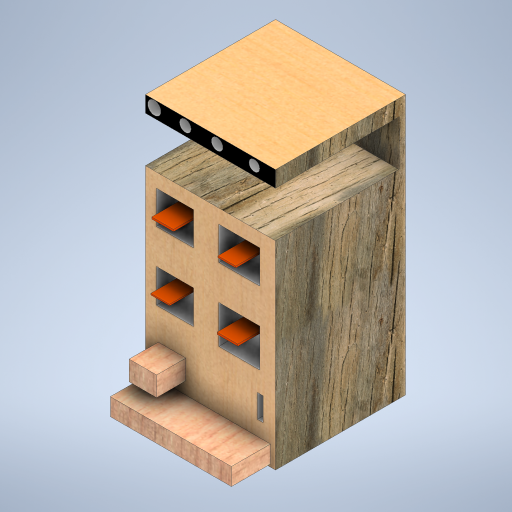
# Autodesk Inventor part: fff
Saved by Autodesk Inventor 2023 (Build 270158000, 158)
## iProperties
Created: 2022-06-05
Part Number: fff
Material: Generic
Document SubType Name: Modeling
Designer: Tushar
Density: 1 g/cm^3
Appearance: Default
Author: Tushar
Autodesk Inventor part; units mm, degrees
ref_plane "YZ Plane" through (0, 0, 0) normal (1, 0, 0) x (0, 1, 0)
ref_plane "XZ Plane" through (0, 0, 0) normal (0, 1, 0) x (-1, 0, 0)
ref_plane "XY Plane" through (0, 0, 0) normal (0, 0, 1) x (1, 0, 0)
sketch "Sketch1" plane through (0, 0, 0) normal (0, 1, 0) x (-1, 0, 0)
  line L0 (17.4506, 75.8516) -> (-84.1494, 75.8516)
  line L1 (-84.1494, 75.8516) -> (-84.1494, -25.7484)
  line L2 (-84.1494, -25.7484) -> (17.4506, -25.7484)
  line L3 (17.4506, -25.7484) -> (17.4506, 75.8516)
  point P0 (0, 0)
  dimension "d0" = 101.6
  dimension "d1" = 101.6
  constraints: 8 end point, 2 parallel, 1 horizontal, 1 perpendicular
  measures "d0" distance of L2.end L0.start
  measures "d1" distance of L1.end L2.end
extrude "Extrusion1" add sketch "Sketch1" along normal blind 203.2
sketch "Sketch2" plane through (-17.4506, 0, 75.8516) normal (0, 0, 1) x (1, 0, 0)
  line L0 (0, 0) -> (0, 203.2) projected
  line L1 (101.6, 0) -> (101.6, 203.2) projected
  line L2 (0, 190.6053) -> (101.6, 190.6053)
  line L3 (101.6, 190.6053) -> (101.6, 155.0988)
  line L4 (101.6, 155.0988) -> (0, 155.0988)
  line L5 (0, 155.0988) -> (0, 190.6053)
  point P0 (17.4506, 0)
  point P1 (0, 155.0988)
  point P2 (101.6, 190.6053)
  constraints: 8 end point, 2 parallel, 2 point on line, 1 horizontal, 1 perpendicular
extrude "Extrusion2" cut sketch "Sketch2" against normal blind 96.52
sketch "Sketch3" plane through (-17.4506, 203.2, 75.8516) normal (0, 0, 1) x (1, 0, 0)
  circle A0 centre (6.9601, -5.4934) radius 5.1747
  circle A1 centre (31.169, -5.4934) radius 4.519
  circle A2 centre (56.0236, -5.4934) radius 4.519
  circle A3 centre (85.0743, -5.4934) radius 4.1962
  point P0 (17.4506, -203.2)
  constraints: 4 centre point
extrude "Extrusion3" cut sketch "Sketch3" against normal blind 8.89
sketch "Sketch4" plane through (-17.4506, 0, 75.8516) normal (0, 0, 1) x (1, 0, 0)
  line L0 (8.574, 144.124) -> (37.6248, 144.124)
  line L1 (37.6248, 144.124) -> (37.6248, 118.3011)
  line L2 (37.6248, 118.3011) -> (8.574, 118.3011)
  line L3 (8.574, 118.3011) -> (8.574, 144.124)
  line L4 (57.3147, 144.124) -> (89.2705, 144.124)
  line L5 (89.2705, 144.124) -> (89.2705, 118.3011)
  line L6 (89.2705, 118.3011) -> (57.3147, 118.3011)
  line L7 (57.3147, 118.3011) -> (57.3147, 144.124)
  line L8 (8.574, 91.1871) -> (37.6248, 91.1871)
  line L9 (37.6248, 91.1871) -> (37.6248, 65.0414)
  line L10 (37.6248, 65.0414) -> (8.574, 65.0414)
  line L11 (8.574, 65.0414) -> (8.574, 91.1871)
  line L12 (57.3147, 91.1871) -> (89.2705, 91.1871)
  line L13 (89.2705, 91.1871) -> (89.2705, 61.4908)
  line L14 (89.2705, 61.4908) -> (57.3147, 61.4908)
  line L15 (57.3147, 61.4908) -> (57.3147, 91.1871)
  point P0 (17.4506, 0)
  constraints: 32 end point, 8 parallel, 7 point on line, 4 horizontal, 4 perpendicular
extrude "Extrusion4" cut sketch "Sketch4" against normal blind 38.1
sketch "Sketch5" plane through (-17.4506, 0, 75.8516) normal (0, 0, 1) x (1, 0, 0)
  line L0 (87.4727, 45.3482) -> (87.4727, 27.2761)
  line L1 (87.4727, 27.2761) -> (91.8686, 27.2761)
  line L2 (91.8686, 27.2761) -> (91.8686, 45.3482)
  line L3 (91.8686, 45.3482) -> (87.4727, 45.3482)
  point P0 (17.4506, 0)
  constraints: 8 end point, 3 perpendicular, 1 vertical
extrude "Extrusion5" cut sketch "Sketch5" against normal blind 25.4
sketch "Sketch6" plane through (-17.4506, 0, 75.8516) normal (0, 0, 1) x (1, 0, 0)
  line L0 (3.0866, 15.6551) -> (97.663, 15.6551)
  line L1 (97.663, 15.6551) -> (97.663, 2.0981)
  line L2 (97.663, 2.0981) -> (3.0866, 2.0981)
  line L3 (3.0866, 2.0981) -> (3.0866, 15.6551)
  point P0 (17.4506, 0)
  constraints: 8 end point, 2 parallel, 1 horizontal, 1 perpendicular
extrude "Extrusion6" add sketch "Sketch6" along normal blind 30.48
sketch "Sketch7" plane through (-17.4506, 0, 75.8516) normal (0, 0, 1) x (1, 0, 0)
  line L0 (10.1224, 40.7313) -> (31.5958, 40.7313)
  line L1 (31.5958, 40.7313) -> (31.5958, 25.3932)
  line L2 (31.5958, 25.3932) -> (10.1224, 25.3932)
  line L3 (10.1224, 25.3932) -> (10.1224, 40.7313)
  point P0 (17.4506, 0)
  constraints: 8 end point, 2 parallel, 1 horizontal, 1 perpendicular
extrude "Extrusion7" add sketch "Sketch7" along normal blind 22.86
sketch "Sketch8" plane through (-17.4506, 0, 37.7516) normal (0, 0, 1) x (1, 0, 0)
  line L0 (18.3983, 134.6076) -> (29.055, 134.6076)
  line L1 (29.055, 134.6076) -> (29.055, 130.1851)
  line L2 (29.055, 130.1851) -> (18.3983, 130.1851)
  line L3 (18.3983, 130.1851) -> (18.3983, 134.6076)
  point P0 (17.4506, 0)
  constraints: 8 end point, 2 parallel, 1 horizontal, 1 perpendicular
extrude "Extrusion8" add sketch "Sketch8" along normal blind 22.86
sketch "Sketch9" plane through (-17.4506, 0, 37.7516) normal (0, 0, 1) x (1, 0, 0)
  line L0 (68.4801, 134.1332) -> (78.7235, 134.1332)
  line L1 (78.7235, 134.1332) -> (78.7235, 130.0548)
  line L2 (78.7235, 130.0548) -> (68.4801, 130.0548)
  line L3 (68.4801, 130.0548) -> (68.4801, 134.1332)
  point P0 (17.4506, 0)
  constraints: 8 end point, 2 parallel, 1 horizontal, 1 perpendicular
extrude "Extrusion9" add sketch "Sketch9" along normal blind 22.86
sketch "Sketch10" plane through (-17.4506, 0, 37.7516) normal (0, 0, 1) x (1, 0, 0)
  line L0 (16.1934, 82.4203) -> (27.2154, 82.4203)
  line L1 (27.2154, 82.4203) -> (27.2154, 79.0146)
  line L2 (27.2154, 79.0146) -> (16.1934, 79.0146)
  line L3 (16.1934, 79.0146) -> (16.1934, 82.4203)
  point P0 (17.4506, 0)
  constraints: 8 end point, 2 parallel, 1 horizontal, 1 perpendicular
extrude "Extrusion10" add sketch "Sketch10" along normal blind 22.86
sketch "Sketch11" plane through (-17.4506, 0, 37.7516) normal (0, 0, 1) x (1, 0, 0)
  line L0 (67.5137, 81.9751) -> (79.9385, 81.9751)
  line L1 (79.9385, 81.9751) -> (79.9385, 78.1143)
  line L2 (79.9385, 78.1143) -> (67.5137, 78.1143)
  line L3 (67.5137, 78.1143) -> (67.5137, 81.9751)
  point P0 (17.4506, 0)
  constraints: 8 end point, 2 parallel, 1 horizontal, 1 perpendicular
extrude "Extrusion11" add sketch "Sketch11" along normal blind 22.86
sketch "Sketch12" plane through (-17.4506, 0, 60.6116) normal (0, 0, 1) x (1, 0, 0)
  line L0 (15.1277, 133.0839) -> (32.1051, 133.0839)
  line L1 (32.1051, 133.0839) -> (32.1051, 131.5664)
  line L2 (32.1051, 131.5664) -> (15.1277, 131.5664)
  line L3 (15.1277, 131.5664) -> (15.1277, 133.0839)
  point P0 (17.4506, 0)
  constraints: 8 end point, 2 parallel, 1 horizontal, 1 perpendicular
extrude "Extrusion12" add sketch "Sketch12" along normal blind 25.4
sketch "Sketch13" plane through (-17.4506, 0, 60.6116) normal (0, 0, 1) x (1, 0, 0)
  line L0 (66.7886, 132.615) -> (80.7539, 132.615)
  line L1 (80.7539, 132.615) -> (80.7539, 131.3454)
  line L2 (80.7539, 131.3454) -> (66.7886, 131.3454)
  line L3 (66.7886, 131.3454) -> (66.7886, 132.615)
  point P0 (17.4506, 0)
  constraints: 8 end point, 2 parallel, 1 horizontal, 1 perpendicular
extrude "Extrusion13" add sketch "Sketch13" along normal blind 25.4
sketch "Sketch14" plane through (-17.4506, 0, 60.6116) normal (0, 0, 1) x (1, 0, 0)
  line L0 (14.3022, 80.9529) -> (29.0306, 80.9529)
  line L1 (29.0306, 80.9529) -> (29.0306, 79.8856)
  line L2 (29.0306, 79.8856) -> (14.3022, 79.8856)
  line L3 (14.3022, 79.8856) -> (14.3022, 80.9529)
  point P0 (17.4506, 0)
  constraints: 8 end point, 2 parallel, 1 horizontal, 1 perpendicular
extrude "Extrusion14" add sketch "Sketch14" along normal blind 25.4
sketch "Sketch15" plane through (-17.4506, 0, 60.6116) normal (0, 0, 1) x (1, 0, 0)
  line L0 (66.065, 80.6327) -> (82.2876, 80.6327)
  line L1 (82.2876, 80.6327) -> (82.2876, 79.1385)
  line L2 (82.2876, 79.1385) -> (66.065, 79.1385)
  line L3 (66.065, 79.1385) -> (66.065, 80.6327)
  point P0 (17.4506, 0)
  constraints: 8 end point, 2 parallel, 1 horizontal, 1 perpendicular
extrude "Extrusion15" add sketch "Sketch15" along normal blind 25.4
sketch "Sketch16" plane through (-17.4506, 155.0988, 75.8516) normal (0, 1, 0) x (1, 0, 0)
  point P0 (17.4506, 75.8516)
body "Solid1"
